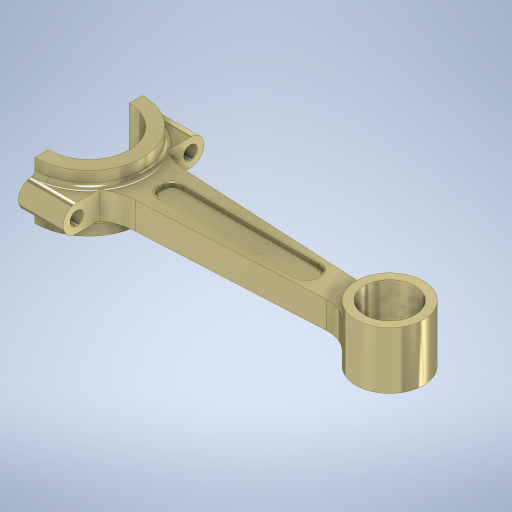
# Autodesk Inventor part: connecting rod
Saved by Autodesk Inventor 2023 (Build 270158000, 158)
## iProperties
Created: 2023-10-21
Part Number: connecting rod
Material: Gold
Document SubType Name: Modeling
Designer: Beatrice
Density: 19.3 g/cm^3
Appearance: Gold - Metal
Author: Beatrice
Autodesk Inventor part; units mm, degrees
ref_plane "YZ Plane" through (0, 0, 0) normal (1, 0, 0) x (0, 1, 0)
ref_plane "XZ Plane" through (0, 0, 0) normal (0, 1, 0) x (-1, 0, 0)
sketch "Sketch1" plane through (0, 0, 0) normal (0, 0, 1) x (1, 0, 0)
  circle A0 centre (0, 0) radius 22.5
  circle A1 centre (0, 0) radius 16.9
  arc A2 (-201.2, -27) -> (-201.2, 27) centre (-201.2, 0) ccw
  arc A3 (-201.2, -36) -> (-201.2, 36) centre (-201.2, 0) ccw
  line L0 (-169.9368, 17.8497) -> (-20.1556, 10)
  line L1 (-169.9368, -17.8497) -> (-20.1556, -10)
  line L2 (-245.94, 0) -> (67.24, 0) construction
  line L3 (-201.2, -36) -> (-201.2, -27)
  line L4 (-201.2, 27) -> (-201.2, 36)
  dimension "d0" = 45
  dimension "d1" = 33.8
  dimension "d2" = 54
  dimension "d3" = 72
  dimension "d4" = 201.2
  dimension "d5" = 6
  dimension "d6" = 20
  constraints: 8 end point, 8 point on circle, 5 coincident, 4 centre point, 4 vertical alignment, 2 vertical, 1 horizontal alignment, 1 other
  measures "d0" diameter of A0
  measures "d1" diameter of A1
  measures "d2" diameter of A2
  measures "d3" diameter of A3
  measures "d4" distance of point (0, 0) A2.centre
  measures "d5" angle of L1 L0
  measures "d6" distance of L1.end L0.end
extrude "Extrusion1" add sketch "Sketch1" along normal mid plane 38 contours A0 | A3 L3 A2 L4
sketch "Sketch2" plane through (0, 0, 0) normal (0, 0, 1) x (1, 0, 0)
  line L0 (-169.9368, 17.8497) -> (-20.1556, 10) projected
  line L1 (-169.9368, -17.8497) -> (-20.1556, -10) projected
  line L2 (-201.2, 27) -> (-201.2, 36) projected
  arc A0 (-201.2, -36) -> (-201.2, 36) centre (-201.2, 0) ccw projected
  line L3 (-201.2, -36) -> (-201.2, -27) projected
  arc A1 (-201.2, -27) -> (-201.2, 27) centre (-201.2, 0) ccw projected
  circle A2 centre (0, 0) radius 16.9 projected
  circle A3 centre (0, 0) radius 22.5 projected
extrude "Extrusion2" add sketch "Sketch2" along normal mid plane 18 contours L0 A3 L1 A0
sketch "Sketch3" plane through (0, 0, 9) normal (0, 0, 1) x (1, 0, 0)
  arc A0 (-201.2, -27) -> (-201.2, 27) centre (-201.2, 0) ccw construction
  circle A1 centre (0, 0) radius 16.9 construction
  line L0 (-201.2, 0) -> (0, 0) construction
  line L1 (-55.6, 8) -> (-145.6, 8)
  line L2 (-145.6, 8) -> (-145.6, -8) construction
  line L3 (-145.6, -8) -> (-55.6, -8)
  line L4 (-55.6, -8) -> (-55.6, 8) construction
  line L5 (-55.6, 8) -> (-145.6, -8) construction
  line L6 (-145.6, 8) -> (-55.6, -8) construction
  arc A2 (-145.6, 8) -> (-145.6, -8) centre (-145.6, 0) ccw
  arc A3 (-55.6, -8) -> (-55.6, 8) centre (-55.6, 0) ccw
  point P0 (-100.6, 0)
  dimension "d11" = 90
  dimension "d12" = 8
  constraints: 14 end point, 6 midpoint, 4 point on circle, 2 centre point, 2 horizontal, 2 parallel, 1 perpendicular
  measures "d11" distance of L1.start L1.end
  measures "d12" radius of A3
extrude "Extrusion3" cut sketch "Sketch3" against normal blind 4
mirror "Mirror1" about plane through (0, 0, 0) normal (0, 0, 1) of "Extrusion3"
fillet "Fillet1" radius 1 8 edges at (-47.6, 0, 9) (-100.6, -8, 9) (-153.6, 0, 9) (-100.6, 8, 9) (-100.6, 8, -9) (-153.6, 0, -9) (-100.6, -8, -9) (-47.6, 0, -9)
fillet "Fillet2" radius 1 8 edges at (-100.6, 8, 5) (-47.6, 0, 5) (-100.6, -8, 5) (-153.6, 0, 5) (-153.6, 0, -5) (-100.6, 8, -5) (-47.6, 0, -5) (-100.6, -8, -5)
fillet "Fillet3" radius 40 2 edges at (-169.9368, -17.8497, 0) (-169.9368, 17.8497, 0)
fillet "Fillet3" radius 22.5 2 edges at (-20.1556, -10, 0) (-20.1556, 10, 0)
ref_plane "Work Plane1" through (-171.2, 27, 19) normal (-1, 0, 0) x (0, 0, 1)
sketch "Sketch4" plane through (-171.2, 27, 19) normal (-1, 0, 0) x (0, 0, 1)
  line L0 (-10, -65) -> (-28, -65) construction
  line L1 (-28, -65) -> (-28, 11)
  line L2 (-28, 11) -> (-10, 11) construction
  line L3 (-10, 11) -> (-10, -65)
  line L4 (-10, -65) -> (-28, 11) construction
  line L5 (-28, -65) -> (-10, 11) construction
  arc A0 (-10, 11) -> (-28, 11) centre (-19, 11) ccw
  arc A1 (-28, -65) -> (-10, -65) centre (-19, -65) ccw
  point P0 (-19, -27)
  dimension "d20" = 76
  dimension "d21" = 9
  constraints: 12 end point, 4 point on circle, 3 midpoint, 2 centre point, 2 parallel, 1 equal radius, 1 horizontal, 1 perpendicular
  measures "d20" distance of L2.end L0.start
  measures "d21" radius of A1
extrude "Extrusion4" add sketch "Sketch4" along normal up to surface (30 mm away)
sketch "Sketch5" plane through (-201.2, -36, -19) normal (-1, 0, 0) x (0, 0, 1)
  arc A0 (28, 74) -> (10, 74) centre (19, 74) ccw projected
  circle A1 centre (19, 74) radius 4.5
  circle A2 centre (19, -2) radius 4.5
  arc A3 (10, -2) -> (28, -2) centre (19, -2) ccw projected
  point P0 (19, 36)
  dimension "d24" = 9
  dimension "d25" = 9
  constraints: 2 centre point, 1 coincident, 1 concentric
  measures "d24" diameter of A1
  measures "d25" diameter of A2
extrude "Extrusion5" cut sketch "Sketch5" against normal through all
fillet "Fillet4" radius 3 2 edges at (-165.2, 0, 9) (-165.2, 0, -9)
sketch "Sketch6" plane through (-201.2, 0, 9) normal (0, 0, 1) x (1, 0, 0)
  arc A0 (0, -27) -> (0, 27) centre (0, 0) ccw projected
  line L0 (0, 27) -> (0, -27) projected
  point P0 (201.2, 0)
extrude "Extrusion6" cut sketch "Sketch6" against normal through all
body "Solid1"
